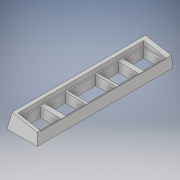
# Autodesk Inventor part: FullConsole
Saved by Autodesk Inventor 2019 (Build 230136000, 136)
## iProperties
Created: 2019-01-04
Part Number: FullConsole
Material: Generic
Document SubType Name: Modeling
Designer: james
Density: 1 g/cm^3
Appearance: Default
Author: james
Autodesk Inventor part; units mm, degrees
ref_plane "YZ Plane" through (0, 0, 0) normal (1, 0, 0) x (0, 1, 0)
ref_plane "XZ Plane" through (0, 0, 0) normal (0, 1, 0) x (-1, 0, 0)
ref_plane "XY Plane" through (0, 0, 0) normal (0, 0, 1) x (1, 0, 0)
sketch "Sketch4" plane through (0, 0, 0) normal (0, 0, 1) x (1, 0, 0)
  line L0 (-144.3789, 43.7906) -> (-144.3789, -108.6094)
  line L1 (-144.3789, -108.6094) -> (160.4211, -108.6094)
  line L2 (160.4211, -108.6094) -> (160.4211, -7.0094)
  line L3 (160.4211, -7.0094) -> (-144.3789, 43.7906)
  point P0 (0, 0)
  dimension "d6" = 304.8
  dimension "d7" = 152.4
  dimension "d8" = 101.6
  constraints: 8 end point, 2 perpendicular, 1 vertical
  measures "d6" distance of L0.end L1.end
  measures "d7" distance of L0.start L0.end
  measures "d8" distance of L1.end L2.end
extrude "Body" add sketch "Sketch4" along normal blind 1371.6
sketch "Sketch5" plane through (160.4211, -108.6094, 0) normal (1, 0, 0) x (0, 0, -1)
  line L0 (-1371.6, 0) -> (-1371.6, 101.6) projected
  line L1 (0, 0) -> (-1371.6, 0) projected
  line L2 (-1371.6, 0) -> (-1318.7374, 299.7986)
  line L3 (-1318.7374, 299.7986) -> (-1508.9577, 299.7986)
  line L4 (-1371.6, 152.4) -> (-1371.6, 0) projected
  line L5 (-1508.9577, 299.7986) -> (-1371.6, 0)
  point P0 (0, 108.6094)
  dimension "d11" = 10
  constraints: 6 end point, 1 perpendicular
  measures "d11" angle of L2 L0
extrude "LeftBevel" cut sketch "Sketch5" against normal blind 1371.6
sketch "Sketch6" plane through (160.4211, -108.6094, 0) normal (1, 0, 0) x (0, 0, -1)
  line L0 (0, 0) -> (0, 101.6) projected
  line L1 (0, 0) -> (-1371.6, 0) projected
  line L2 (0, 0) -> (-29.2918, 166.1219)
  line L3 (-29.2918, 166.1219) -> (35.444, 166.1219)
  line L4 (35.444, 166.1219) -> (0, 0)
  point P0 (0, 108.6094)
  dimension "d14" = 10
  constraints: 6 end point, 1 parallel
  measures "d14" angle of L2 L0
extrude "RightBevel" [suppressed]
sketch "Sketch7" plane through (0, 0, 1371.6) normal (0, 0, 1) x (1, 0, 0)
  line L0 (-144.3789, 43.7906) -> (-144.3789, -108.6094) projected
  line L1 (-144.3789, -108.6094) -> (-110.1629, 85.4397)
  line L2 (-110.1629, 85.4397) -> (-236.272, 85.4397)
  line L3 (-236.272, 85.4397) -> (-144.3789, -108.6094)
  point P0 (0, 0)
  dimension "d17" = 10
  constraints: 6 end point, 1 horizontal
  measures "d17" angle of L0 L1
extrude "BackBevel" cut sketch "Sketch7" against normal blind 1371.6
sketch "Sketch8" plane through (0, 0, 1371.6) normal (0, 0, 1) x (1, 0, 0)
  line L0 (160.4211, -108.6094) -> (160.4211, -7.0094) projected
  line L1 (-144.3789, -108.6094) -> (160.4211, -108.6094) projected
  line L2 (160.4211, -108.6094) -> (129.3641, 67.5233)
  line L3 (129.3641, 67.5233) -> (267.9679, 67.5233)
  line L4 (267.9679, 67.5233) -> (160.4211, -108.6094)
  point P0 (0, 0)
  dimension "d20" = 10
  constraints: 6 end point, 1 parallel
  measures "d20" angle of L2 L0
extrude "FrontBevel" cut sketch "Sketch8" against normal blind 1371.6
sketch "Sketch9" plane through (-144.3789, -108.6094, 0) normal (0, -1, 0) x (1, 0, 0)
  line L0 (286.893, 1320.8) -> (58.293, 1320.8)
  line L1 (58.293, 1320.8) -> (58.293, 50.8)
  line L2 (58.293, 50.8) -> (286.893, 50.8)
  line L3 (286.893, 50.8) -> (286.893, 1320.8)
  line L4 (304.8, 0) -> (304.8, 1371.6) projected
  line L5 (0, 0) -> (304.8, 0) projected
  line L6 (0, 1371.6) -> (304.8, 1371.6) projected
  point P0 (144.3789, 0)
  dimension "d24" = 228.6
  dimension "d25" = 17.907
  dimension "d26" = 50.8
  dimension "d31" = 50.8
  constraints: 8 end point, 2 parallel, 1 horizontal, 1 perpendicular
  measures "d24" distance of L1.end L2.end
  measures "d25" distance between parallel lines of L3 L4
  measures "d26" distance between parallel lines of L5 L2
  measures "d31" distance between parallel lines of L6 L0
extrude "BottomEx" add sketch "Sketch9" against normal blind 152.4
sketch "Sketch10" plane through (-144.3789, 43.7906, 0) normal (0, 1, 0) x (1, 0, 0)
  line L0 (58.293, -1320.8) -> (286.893, -1320.8) projected
  line L1 (286.893, -1320.8) -> (286.893, -50.8) projected
  line L2 (286.893, -50.8) -> (58.293, -50.8) projected
  line L3 (58.293, -50.8) -> (58.293, -1320.8) projected
  line L4 (58.293, -50.8) -> (286.893, -50.8) projected
  line L5 (286.893, -50.8) -> (58.293, -50.8)
  line L6 (58.293, -50.8) -> (58.293, -1320.8)
  line L7 (58.293, -1320.8) -> (286.893, -1320.8)
  line L8 (286.893, -1320.8) -> (286.893, -50.8)
  point P0 (144.3789, 0)
  point P1 (26.1051, -50.8)
  constraints: 8 end point, 2 parallel, 1 horizontal, 1 perpendicular
extrude "Extrusion8" cut sketch "Sketch10" against normal blind 57.15
sketch "Sketch11" plane through (-144.3789, -13.3594, 0) normal (0, 1, 0) x (1, 0, 0)
  line L0 (70.993, -266.7) -> (274.193, -266.7)
  line L1 (274.193, -266.7) -> (274.193, -63.5)
  line L2 (274.193, -63.5) -> (70.993, -63.5)
  line L3 (70.993, -63.5) -> (70.993, -266.7)
  line L4 (58.293, -1320.8) -> (58.293, -50.8) projected
  line L5 (58.293, -50.8) -> (286.893, -50.8) projected
  point P0 (144.3789, 0)
  dimension "d32" = 203.2
  dimension "d33" = 203.2
  dimension "d34" = 12.7
  dimension "d35" = 12.7
  constraints: 8 end point, 2 parallel, 1 horizontal, 1 perpendicular
  measures "d32" distance of L2.end L0.start
  measures "d33" distance of L1.end L2.end
  measures "d34" distance between parallel lines of L3 L4
  measures "d35" distance between parallel lines of L5 L2
extrude "Extrusion9" cut sketch "Sketch11" against normal blind 174.625
sketch "Sketch12" plane through (-144.3789, -13.3594, 0) normal (0, 1, 0) x (1, 0, 0)
  line L0 (58.293, -1320.8) -> (58.293, -50.8) projected
  line L1 (286.893, -1320.8) -> (58.293, -1320.8) projected
  line L2 (70.993, -1308.1) -> (274.193, -1308.1)
  line L3 (274.193, -1308.1) -> (274.193, -1104.9)
  line L4 (274.193, -1104.9) -> (70.993, -1104.9)
  line L5 (70.993, -1104.9) -> (70.993, -1308.1)
  point P0 (144.3789, 0)
  dimension "d38" = 203.2
  dimension "d39" = 203.2
  dimension "d40" = 12.7
  dimension "d41" = 12.7
  constraints: 8 end point, 2 parallel, 1 horizontal, 1 perpendicular
  measures "d38" distance of L3.end L4.end
  measures "d39" distance of L2.end L3.end
  measures "d40" distance between parallel lines of L2 L1
  measures "d41" distance between parallel lines of L0 L5
extrude "Extrusion10" cut sketch "Sketch12" against normal blind 166.6875
sketch "Sketch13" plane through (-144.3789, -13.3594, 0) normal (0, 1, 0) x (1, 0, 0)
  line L0 (70.993, -266.7) -> (70.993, -63.5) projected
  line L1 (70.993, -266.7) -> (274.193, -266.7) projected
  line L2 (274.193, -266.7) -> (70.993, -266.7) projected
  line L3 (274.193, -266.7) -> (70.993, -266.7) projected
  line L4 (70.993, -317.5) -> (274.193, -317.5)
  line L5 (274.193, -317.5) -> (274.193, -520.7)
  line L6 (274.193, -520.7) -> (70.993, -520.7)
  line L7 (70.993, -520.7) -> (70.993, -317.5)
  point P0 (144.3789, 0)
  dimension "d44" = 0
  dimension "d45" = 50.8
  dimension "d46" = 203.2
  dimension "d47" = 203.2
  constraints: 8 end point, 2 parallel, 1 horizontal, 1 perpendicular
  measures "d44" distance between parallel lines of L0 L7
  measures "d45" distance between parallel lines of L2 L4
  measures "d46" distance of L5.end L6.end
  measures "d47" distance of L4.end L5.end
extrude "Extrusion11" cut sketch "Sketch13" against normal blind 166.6875
sketch "Sketch14" plane through (-144.3789, -13.3594, 0) normal (0, 1, 0) x (1, 0, 0)
  line L0 (70.993, -1308.1) -> (70.993, -1104.9) projected
  line L1 (70.993, -1104.9) -> (274.193, -1104.9) projected
  line L2 (70.993, -1054.1) -> (274.193, -1054.1)
  line L3 (274.193, -1054.1) -> (274.193, -850.9)
  line L4 (274.193, -850.9) -> (70.993, -850.9)
  line L5 (70.993, -850.9) -> (70.993, -1054.1)
  point P0 (144.3789, 0)
  dimension "d50" = 0
  dimension "d51" = 50.8
  dimension "d52" = 203.2
  dimension "d53" = 203.2
  constraints: 8 end point, 2 parallel, 1 horizontal, 1 perpendicular
  measures "d50" distance between parallel lines of L0 L5
  measures "d51" distance between parallel lines of L1 L2
  measures "d52" distance of L3.end L4.end
  measures "d53" distance of L2.end L3.end
extrude "Extrusion12" cut sketch "Sketch14" against normal blind 166.6875
sketch "Sketch15" plane through (-144.3789, -13.3594, 0) normal (0, 1, 0) x (1, 0, 0)
  line L0 (70.993, -825.5) -> (274.193, -825.5)
  line L1 (274.193, -825.5) -> (274.193, -546.1)
  line L2 (274.193, -546.1) -> (70.993, -546.1)
  line L3 (70.993, -546.1) -> (70.993, -825.5)
  line L4 (70.993, -520.7) -> (70.993, -317.5) projected
  line L5 (274.193, -520.7) -> (70.993, -520.7) projected
  line L6 (70.993, -850.9) -> (274.193, -850.9) projected
  point P0 (144.3789, 0)
  dimension "d56" = 279.4
  dimension "d57" = 203.2
  dimension "d58" = 0
  dimension "d59" = 25.4
  dimension "d60" = 25.4
  constraints: 8 end point, 2 parallel, 1 horizontal, 1 perpendicular
  measures "d56" distance of L2.end L0.start
  measures "d57" distance of L1.end L2.end
  measures "d58" distance between parallel lines of L4 L3
  measures "d59" distance between parallel lines of L5 L2
  measures "d60" distance between parallel lines of L6 L0
extrude "Extrusion13" cut sketch "Sketch15" against normal blind 166.6875
sketch "Sketch16" plane through (-144.3789, -108.6094, 0) normal (-0.9848078, 0.1736482, 0) x (0, 0, 1)
  line L0 (297.688, 126.8744) -> (1073.912, 126.8744)
  line L1 (1073.912, 126.8744) -> (1073.912, 29.8464)
  line L2 (1073.912, 29.8464) -> (297.688, 29.8464)
  line L3 (297.688, 29.8464) -> (297.688, 126.8744)
  line L4 (0, 0) -> (0, 150.3331) projected
  point P0 (0, 132.0305)
  dimension "d63" = 97.028
  dimension "d64" = 776.224
  dimension "d65" = 297.688
  constraints: 8 end point, 2 parallel, 1 horizontal, 1 perpendicular
  measures "d63" distance of L0.end L1.end
  measures "d64" distance of L0.start L0.end
  measures "d65" distance between parallel lines of L4 L3
extrude "Extrusion14" cut sketch "Sketch16" against normal blind 15.24
body "Solid2"
